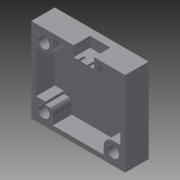
# Autodesk Inventor part: case_top
Saved by Autodesk Inventor 2015 SP1 (Build 190203100, 203)
## iProperties
Created: 2015-12-01
Part Number: case_top
Material: Polycarbonate, Clear
Document SubType Name: Modeling
Designer: User
Density: 1.2 g/cm^3
Appearance: Polycarbonate - Clear
Mass: 7.45 g
Surface Area: 58.0738 cm^2
Volume: 6.20834 cm^3
Author: User
Autodesk Inventor part; units mm, degrees
note: some values were not read from the file. Chosen so that the rebuilt part matches the saved one: sketch regions of "Выдавливание2".
ref_plane "YZ Plane" through (0, 0, 0) normal (1, 0, 0) x (0, 1, 0)
ref_plane "XZ Plane" through (0, 0, 0) normal (0, 1, 0) x (-1, 0, 0)
ref_plane "XY Plane" through (0, 0, 0) normal (0, 0, 1) x (1, 0, 0)
sketch "Эскиз1" plane through (0, 0, 0) normal (0, 1, 0) x (-1, 0, 0)
  line L0 (18, -16) -> (-18, -16)
  line L1 (-18, -16) -> (-18, 16)
  line L2 (-18, 16) -> (18, 16)
  line L3 (18, 16) -> (18, -16)
  line L4 (0, -25.5623) -> (0, 25.8016) projected
  line L5 (28.3623, 0) -> (-28.6016, 0) projected
  line L6 (14.82, -12.82) -> (-14.82, -12.82)
  line L7 (-14.82, -12.82) -> (-14.82, 12.82)
  line L8 (-14.82, 12.82) -> (14.82, 12.82)
  line L9 (14.82, 12.82) -> (14.82, -12.82)
  circle A0 centre (14.82, -12.82) radius 2.5
  circle A1 centre (14.82, 12.82) radius 2.5
  circle A2 centre (-14.82, 12.82) radius 2.5
  circle A3 centre (-14.82, -12.82) radius 2.5
  arc A4 (11.9634, -10.02) -> (14.12, -8.8817) centre (14.82, -12.82) ccw
  circle A5 centre (-14.82, -12.82) radius 4
  arc A6 (14.12, 8.8817) -> (12.7129, 9.42) centre (14.82, 12.82) ccw
  arc A7 (-11.0303, 14.1) -> (-16.6, 9.2379) centre (-14.82, 12.82) ccw
  line L10 (14.12, -10.02) -> (1.12, -10.02)
  line L11 (1.12, -10.02) -> (1.12, 9.42)
  line L12 (1.12, 9.42) -> (14.12, 9.42)
  line L13 (14.12, 9.42) -> (14.12, -10.02)
  line L14 (-9.6, 7.9) -> (-16.6, 7.9)
  line L15 (-16.6, 7.9) -> (-16.6, 14.1)
  line L16 (-16.6, 14.1) -> (-9.6, 14.1)
  line L17 (-9.6, 14.1) -> (-9.6, 7.9)
  line L18 (-11.0303, 14.1) -> (-16.6, 14.1)
  line L19 (14.12, 8.8817) -> (14.12, 9.42)
  line L20 (14.12, -8.8817) -> (14.12, -10.02)
  line L21 (11.9634, -10.02) -> (14.12, -10.02)
  circle A8 centre (-13.034, 10.913) radius 1.5
  circle A9 centre (-13.034, 10.913) radius 1.25
  line L22 (20, -18) -> (-20, -18)
  line L23 (-20, -18) -> (-20, 18)
  line L24 (-20, 18) -> (20, 18)
  line L25 (20, 18) -> (20, -18)
  line L26 (-10.82, -12.82) -> (-10.82, -16)
  line L27 (-14.82, -8.82) -> (-18, -8.82)
  line L28 (10.82, -12.82) -> (10.82, -16)
  line L29 (14.82, -8.82) -> (18, -8.82)
  line L30 (14.82, 8.82) -> (18, 8.82)
  line L31 (10.82, 12.82) -> (10.82, 16)
  line L32 (-18, 8.82) -> (-16.6, 8.82)
  line L33 (-10.82, 16) -> (-10.82, 14.1)
  line L34 (-10.82, 14.1) -> (-11.0303, 14.1)
  line L35 (-16.6, 9.2379) -> (-16.6, 8.82)
  line L36 (3.5, 16) -> (3.5, 12.6)
  line L37 (3.5, 12.6) -> (-8.2, 12.6)
  line L38 (-8.2, 12.6) -> (-8.2, 16)
  line L39 (-6.7, 18) -> (-6.7, 13.6)
  line L40 (-6.7, 13.6) -> (2, 13.6)
  line L41 (2, 13.6) -> (2, 18)
  point P0 (0, 0)
  dimension "d0" = 36
  dimension "d1" = 32
  dimension "d2" = 3.18
  dimension "d3" = 3.18
  dimension "d4" = 3.18
  dimension "d5" = 3.18
  dimension "d6" = 5
  dimension "d7" = 5
  dimension "d8" = 5
  dimension "d9" = 5
  dimension "d10" = 8
  dimension "d11" = 8
  dimension "d12" = 8
  dimension "d13" = 8
  dimension "d14" = 2.8
  dimension "d15" = 0.7
  dimension "d16" = 3.4
  dimension "d17" = 13
  dimension "d18" = 1.9
  dimension "d19" = 1.4
  dimension "d20" = 7
  dimension "d21" = 6.2
  dimension "d22" = 4.966
  dimension "d23" = 5.087
  dimension "d24" = 3
  dimension "d25" = 2.5
  dimension "d26" = 2
  dimension "d27" = 2
  dimension "d28" = 2
  dimension "d29" = 2
  dimension "d30" = 4
  dimension "d32" = 4
  dimension "d33" = 16
  dimension "d34" = 11.3
  dimension "d35" = 1
  dimension "d36" = 1.5
  dimension "d37" = 1.5
  dimension "d38" = 2.4
  constraints: 80 end point, 27 point on line, 16 perpendicular, 12 point on circle, 11 parallel, 10 centre point, 10 coincident, 5 horizontal, 3 collinear, 3 tangent, 2 vertical, 2 other
  measures "d0" distance of L0.start L0.end
  measures "d1" distance of L0.end L1.end
  measures "d2" distance between parallel lines of L3 L9
  measures "d3" distance between parallel lines of L2 L8
  measures "d4" distance between parallel lines of L1 L7
  measures "d5" distance between parallel lines of L0 L6
  measures "d6" diameter of A0
  measures "d7" diameter of A1
  measures "d8" diameter of A2
  measures "d9" diameter of A3
  measures "d10" diameter of A4
  measures "d11" diameter of A5
  measures "d12" diameter of A6
  measures "d13" diameter of A7
  measures "d14" distance between parallel lines of L6 L10
  measures "d15" distance between parallel lines of L9 L13
  measures "d16" distance between parallel lines of L8 L12
  measures "d17" distance of L11.end L12.end
  measures "d18" distance between parallel lines of L2 L16
  measures "d19" distance between parallel lines of L1 L15
  measures "d20" distance of L14.start L14.end
  measures "d21" distance of L16.end L14.start
  measures "d22" distance from line of L1 point (-13.034, 10.913)
  measures "d23" distance from line of L2 point (-13.034, 10.913)
  measures "d24" diameter of A8
  measures "d25" diameter of A9
  measures "d26" distance between parallel lines of L22 L0
  measures "d27" distance between parallel lines of L25 L3
  measures "d28" distance between parallel lines of L2 L24
  measures "d29" distance between parallel lines of L23 L1
  measures "d30" distance between parallel lines of L32 L8
  measures "d32" distance between parallel lines of L33 L7
  measures "d33" distance between parallel lines of L3 L41
  measures "d34" distance between parallel lines of L1 L39
  measures "d35" distance between parallel lines of L37 L40
  measures "d36" distance between parallel lines of L36 L41
  measures "d37" distance between parallel lines of L38 L39
  measures "d38" distance between parallel lines of L40 L2
extrude "Выдавливание1" add sketch "Эскиз1" against normal blind 10 contours L3 A4 L5 L25 L22 L4 L0 | L0 A4 L3 | A4 L0 | L0 A4 L6 A0 L9 L3 | L3 A4 | L0 L28 A4 | A4 L29 L3 | A4 L10 L13 L9 A0 L6 | L4 L22 L23 L5 L1 A5 L0 | A0 L9 L6 | L6 L9 A0 | L3 A6 L2 L41 L24 L25 L5 | L0 A5 L26 | A5 L0 L1 L7 A3 L6 | L6 A3 L7 A5 | L30 A6 L3 | A6 L13 L12 L8 A1 L9 | L9 A1 L8 A6 L2 L3 | A5 L0 | A3 L7 L6 | L6 L7 A3 | A5 L1 L27 | L3 A6 | A1 L8 L9 | L9 L8 A1 | L0 L1 A5 | L23 L24 L39 L2 A7 L1 L5 | L8 L38 L2 L39 L40 L4 | L4 L40 L41 L2 L36 L8 | L1 A5 | A6 L2 L3 | L1 A7 L15 L32 | L2 A6 | L31 L2 A6 | A7 L1 | L1 A7 L2 L16 A2 L15 | A2 L16 L15 | L33 L16 A7 L2 | L1 L2 A7 | L2 A7
extrude "Выдавливание2" add sketch "Эскиз1" against normal blind 2 contours L0 L4 L6 L28 | L6 L4 L5 L11 L10 A4 | L29 L9 L5 L3 | A4 L13 L5 L9 | L0 L26 L6 L4 | L6 A5 L7 L5 L4 | L10 L11 L5 L13 | L5 L9 L30 L3 | L5 L13 A6 L9 | L5 L7 L14 L17 L8 L38 L37 L4 | L4 L37 L36 L8 A6 L12 L11 L5 | L5 L11 L12 L13 | L37 L38 L8 L4 | L4 L8 L36 L37 | L7 L27 L1 L5 | L5 L1 L32 L15 L14 L7 | L8 L38 L2 L39 L40 L4 | L4 L40 L41 L2 L36 L8 | L14 L15 A2 L7 | L7 A2 A8 L8 L17 L14 | L40 L39 L2 L4 | L4 L2 L41 L40 | L8 L17 L16 L33 L2 L38 | L36 L2 L31 L8 | A2 L15 L16 L8 L7 | L7 L8 A2 A8 | L8 A2 L16 L17
extrude "Выдавливание3" add sketch "Эскиз1" against normal blind 3 contours L41 L2 L4 L24 | L40 L39 L2 L4 | L4 L2 L41 L40 | L4 L2 L39 L24
sketch "Эскиз2" plane through (0, -10, 0) normal (0, -1, 0) x (1, 0, 0)
  circle A0 centre (-14.82, 12.82) radius 2.5 projected
  circle A1 centre (-14.82, -12.82) radius 2.5 projected
  circle A2 centre (14.82, 12.82) radius 2.5 projected
  circle A3 centre (14.82, -12.82) radius 2.5 projected
  point P0 (0, 0)
extrude "Выдавливание4" cut sketch "Эскиз2" against normal blind 5 contours A0 | A1 | A3
sketch "Эскиз4" plane through (-2, -10, 13.6) normal (0, 0, 1) x (1, 0, 0)
  line L0 (8.7, 7) -> (0, 7) projected
  line L1 (0, 7) -> (0, 0) projected
  line L2 (8.7, 0) -> (0, 0) projected
  line L3 (8.7, 7) -> (8.7, 0) projected
  line L4 (12.82, 0) -> (-8.82, 0) projected
  line L5 (1.85, 2.5) -> (2.85, 2.5)
  line L6 (2.85, 2.5) -> (2.85, 0)
  line L7 (2.85, 0) -> (1.85, 0)
  line L8 (1.85, 0) -> (1.85, 2.5)
  line L9 (4.35, 7.5527) -> (4.35, -2.1093)
  line L10 (6.85, 2.5) -> (5.85, 2.5)
  line L11 (5.85, 2.5) -> (5.85, 0)
  line L12 (5.85, 0) -> (6.85, 0)
  line L13 (6.85, 0) -> (6.85, 2.5)
  point P0 (2, 10)
  dimension "d66" = 4.35
  dimension "d67" = 1
  dimension "d68" = 2.5
  dimension "d69" = 4
  constraints: 18 end point, 4 symmetric about line, 2 parallel, 1 horizontal, 1 perpendicular, 1 point on line, 1 vertical
  measures "d66" distance between parallel lines of L1 L9
  measures "d67" distance of L5.start L5.end
  measures "d68" distance of L7.end L5.start
  measures "d69" distance between parallel lines of L11 L8
extrude "Выдавливание5" cut sketch "Эскиз4" against normal up to next contours L2 L11 L10 L13 | L2 L8 L5 L6
